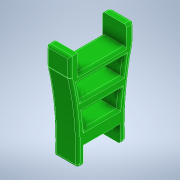
# Autodesk Inventor part: arm_mid_link
Saved by Autodesk Inventor 2022 (Build 260153000, 153)
## iProperties
Created: 2022-04-24
Part Number: arm_mid_link
Material: Generic
Document SubType Name: Modeling
Designer: HP
Density: 1 g/cm^3
Appearance: Dark Green
Author: HP
Autodesk Inventor part; units mm, degrees
ref_plane "YZ Plane" through (0, 0, 0) normal (1, 0, 0) x (0, 1, 0)
ref_plane "XZ Plane" through (0, 0, 0) normal (0, 1, 0) x (-1, 0, 0)
ref_plane "XY Plane" through (0, 0, 0) normal (0, 0, 1) x (1, 0, 0)
sketch "Sketch2" plane through (0, 0, 0) normal (1, 0, 0) x (0, 1, 0)
  line L0 (-7.3755, -15.6467) -> (7.3755, -15.6467)
  line L1 (7.3755, -15.6467) -> (7.3755, 15.6467)
  line L2 (7.3755, 15.6467) -> (-7.3755, 15.6467)
  line L3 (-7.3755, -15.6467) -> (7.3755, 15.6467) construction
  line L4 (7.3755, -15.6467) -> (-7.3755, 15.6467) construction
  line L5 (60.9777, -20.5594) -> (77.0347, -20.5594)
  line L6 (77.0347, 20.5594) -> (60.9777, 20.5594)
  line L7 (60.9777, 20.5594) -> (60.9777, -20.5594)
  line L8 (60.9777, -20.5594) -> (61.2067, -19.973) construction
  line L9 (77.0347, -20.5594) -> (77.0347, -26.8297)
  line L10 (77.0347, -26.8297) -> (60.9777, -26.8297)
  line L11 (77.0347, 20.5594) -> (77.0347, 26.8297)
  line L12 (77.0347, 26.8297) -> (60.9777, 26.8297)
  line L13 (-7.3755, -15.6467) -> (-7.3755, -20.5594)
  line L14 (-7.3755, 15.6467) -> (-7.3755, 20.5594)
  arc A0 (-7.3755, 20.5594) -> (60.9777, 26.8297) centre (5.2184, 258.9699) ccw
  line L15 (105.2893, 0) -> (-40.5688, 0)
  arc A1 (60.9777, -26.8297) -> (-7.3755, -20.5594) centre (5.2184, -258.9699) ccw
  line L16 (18.2679, -14.0216) -> (18.2679, 14.0216)
  line L17 (31.1322, -14.0216) -> (18.2679, 14.0216) construction
  line L18 (18.2679, -14.0216) -> (31.1322, 14.0216) construction
  line L19 (40.8525, -17.2571) -> (40.8525, 17.2571)
  line L20 (53.7613, -17.2571) -> (40.8525, 17.2571) construction
  line L21 (40.8525, -17.2571) -> (53.7613, 17.2571) construction
  line L22 (40.8525, -17.2571) -> (54.5312, -19.3156)
  line L23 (54.5312, -19.3156) -> (54.7625, 19.9339)
  line L24 (54.7625, 19.9339) -> (40.8525, 17.2571)
  line L25 (18.2679, -14.0216) -> (32.0056, -15.9257)
  line L26 (32.0056, -15.9257) -> (32.0056, 15.5546)
  line L27 (32.0056, 15.5546) -> (18.2679, 14.0216)
  point P0 (0, 0)
  point P1 (24.7, 0)
  point P2 (47.3069, 0)
  dimension "d5" = 6.2703
  dimension "d6" = 6.2703
  dimension "d7" = 34.5141
  dimension "d8" = 34.5141
  constraints: 56 end point, 6 midpoint, 4 point on circle, 4 vertical, 3 horizontal, 3 perpendicular, 3 point on line, 2 centre point, 2 parallel, 1 symmetric about line, 1 other
  measures "d5" distance between parallel lines of L10 L5
  measures "d6" distance between parallel lines of L6 L12
  measures "d7" distance of L19.start L19.end
  measures "d8" distance of L21.end L20.start
extrude "Extrusion2" add sketch "Sketch2" along normal blind 20 contours L0 L1 L15 L16 L25 L26 L19 L22 L23 L7 L5 L9 L10 A1 L13 | L1 L2 L14 A0 L12 L11 L6 L7 L15 L23 L24 L19 L26 L27 L16
sketch "Sketch3" plane through (0, 60.9777, -26.8297) normal (0, 0, -1) x (-1, 0, 0)
  point P0 (0, -60.9777)
fillet "Fillet2" radius 2 38 edges at (20, 69.0062, 26.8297) (20, 27.0276, 21.2253) (10, 60.9777, 26.8297) (0, 27.0276, 21.2253) (10, -7.3755, 20.5594) (10, 77.0347, 26.8297) (0, 69.0062, 26.8297) (20, 69.0062, -26.8297) (10, 77.0347, -26.8297) (0, 77.0347, 23.6946) (0, 77.0347, -23.6946) (20, 77.0347, -23.6946) (20, 60.9777, 0) (0, 60.9777, 0) (20, 54.6469, 0.3091) (20, 40.8525, 0) (20, 32.0056, -0.1855) (20, 18.2679, 0) (20, 25.1367, -14.9737) (20, 25.1367, 14.7881) (20, 47.8075, 18.5955) (20, 47.6919, -18.2863) (20, -7.3755, -18.1031) (20, -7.3755, 18.1031) (0, 27.0276, -21.2253) (0, 69.0062, -26.8297) (10, 60.9777, -26.8297) (10, -7.3755, -20.5594) (20, 27.0276, -21.2253) (0, 7.3755, 0) (0, 18.2679, 0) (0, 32.0056, -0.1855) (0, 40.8525, 0) (0, 54.6469, 0.3091) (0, 47.8075, 18.5955) (0, 25.1367, 14.7881) (0, 25.1367, -14.9737) (0, 47.6919, -18.2863)
body "Solid2"
